Autodesk Inventor part; units mm, degrees
(part 3 of 4)
  line L545 (-44.5, 18.2583) -> (-43, 20.8564)
  line L546 (-59, 20.8564) -> (-60.5, 23.4545)
  line L547 (-60.5, 23.4545) -> (-63.5, 23.4545)
  line L548 (-63.5, 23.4545) -> (-65, 20.8564)
  line L549 (-65, 20.8564) -> (-63.5, 18.2583)
  line L550 (-63.5, 18.2583) -> (-60.5, 18.2583)
  line L551 (-60.5, 18.2583) -> (-59, 20.8564)
  line L552 (-75, 20.8564) -> (-76.5, 23.4545)
  line L553 (-76.5, 23.4545) -> (-79.5, 23.4545)
  line L554 (-79.5, 23.4545) -> (-81, 20.8564)
  line L555 (-81, 20.8564) -> (-79.5, 18.2583)
  line L556 (-79.5, 18.2583) -> (-76.5, 18.2583)
  line L557 (-76.5, 18.2583) -> (-75, 20.8564)
  line L558 (-80.5, 30.5263) -> (-83.5, 30.5263)
  line L559 (-83.5, 30.5263) -> (-85, 27.9282)
  line L560 (-85, 27.9282) -> (-83.5, 25.3301)
  line L561 (-83.5, 25.3301) -> (-80.5, 25.3301)
  line L562 (-80.5, 25.3301) -> (-79, 27.9282)
  line L563 (-79, 27.9282) -> (-80.5, 30.5263)
  line L564 (-47, 27.9282) -> (-48.5, 30.5263)
  line L565 (-48.5, 30.5263) -> (-51.5, 30.5263)
  line L566 (-51.5, 30.5263) -> (-53, 27.9282)
  line L567 (-53, 27.9282) -> (-51.5, 25.3301)
  line L568 (-51.5, 25.3301) -> (-48.5, 25.3301)
  line L569 (-48.5, 25.3301) -> (-47, 27.9282)
  line L570 (-67.5, 25.3301) -> (-64.5, 25.3301)
  line L571 (-64.5, 25.3301) -> (-63, 27.9282)
  line L572 (-63, 27.9282) -> (-64.5, 30.5263)
  line L573 (-64.5, 30.5263) -> (-67.5, 30.5263)
  line L574 (-67.5, 30.5263) -> (-69, 27.9282)
  line L575 (-69, 27.9282) -> (-67.5, 25.3301)
  line L576 (-39.5, 37.4545) -> (-41, 34.8564)
  line L577 (-41, 34.8564) -> (-39.5, 32.2583)
  line L578 (-39.5, 32.2583) -> (-36.5, 32.2583)
  line L579 (-36.5, 32.2583) -> (-35, 34.8564)
  line L580 (-35, 34.8564) -> (-36.5, 37.4545)
  line L581 (-36.5, 37.4545) -> (-39.5, 37.4545)
  line L582 (-55.5, 32.2583) -> (-52.5, 32.2583)
  line L583 (-52.5, 32.2583) -> (-51, 34.8564)
  line L584 (-51, 34.8564) -> (-52.5, 37.4545)
  line L585 (-52.5, 37.4545) -> (-55.5, 37.4545)
  line L586 (-55.5, 37.4545) -> (-57, 34.8564)
  line L587 (-57, 34.8564) -> (-55.5, 32.2583)
  line L588 (-71.5, 32.2583) -> (-68.5, 32.2583)
  line L589 (-68.5, 32.2583) -> (-67, 34.8564)
  line L590 (-67, 34.8564) -> (-68.5, 37.4545)
  line L591 (-68.5, 37.4545) -> (-71.5, 37.4545)
  line L592 (-71.5, 37.4545) -> (-73, 34.8564)
  line L593 (-73, 34.8564) -> (-71.5, 32.2583)
  line L594 (-15.5, 32.2583) -> (-12.5, 32.2583)
  line L595 (-12.5, 32.2583) -> (-11, 34.8564)
  line L596 (-11, 34.8564) -> (-12.5, 37.4545)
  line L597 (-12.5, 37.4545) -> (-15.5, 37.4545)
  line L598 (-15.5, 37.4545) -> (-17, 34.8564)
  line L599 (-17, 34.8564) -> (-15.5, 32.2583)
  line L600 (-35.5, 25.3301) -> (-32.5, 25.3301)
  line L601 (-32.5, 25.3301) -> (-31, 27.9282)
  line L602 (-31, 27.9282) -> (-32.5, 30.5263)
  line L603 (-32.5, 30.5263) -> (-35.5, 30.5263)
  line L604 (-35.5, 30.5263) -> (-37, 27.9282)
  line L605 (-37, 27.9282) -> (-35.5, 25.3301)
  line L606 (-25, 34.8564) -> (-23.5, 32.2583)
  line L607 (-23.5, 32.2583) -> (-20.5, 32.2583)
  line L608 (-20.5, 32.2583) -> (-19, 34.8564)
  line L609 (-19, 34.8564) -> (-20.5, 37.4545)
  line L610 (-20.5, 37.4545) -> (-23.5, 37.4545)
  line L611 (-23.5, 37.4545) -> (-25, 34.8564)
  line L612 (-7, 27.9282) -> (-8.5, 30.5263)
  line L613 (-8.5, 30.5263) -> (-11.5, 30.5263)
  line L614 (-11.5, 30.5263) -> (-13, 27.9282)
  line L615 (-13, 27.9282) -> (-11.5, 25.3301)
  line L616 (-11.5, 25.3301) -> (-8.5, 25.3301)
  line L617 (-8.5, 25.3301) -> (-7, 27.9282)
  line L618 (-80.5, 44.5263) -> (-83.5, 44.5263)
  line L619 (-83.5, 44.5263) -> (-85, 41.9282)
  line L620 (-85, 41.9282) -> (-83.5, 39.3301)
  line L621 (-83.5, 39.3301) -> (-80.5, 39.3301)
  line L622 (-80.5, 39.3301) -> (-79, 41.9282)
  line L623 (-79, 41.9282) -> (-80.5, 44.5263)
  line L624 (-47, 41.9282) -> (-48.5, 44.5263)
  line L625 (-48.5, 44.5263) -> (-51.5, 44.5263)
  line L626 (-51.5, 44.5263) -> (-53, 41.9282)
  line L627 (-53, 41.9282) -> (-51.5, 39.3301)
  line L628 (-51.5, 39.3301) -> (-48.5, 39.3301)
  line L629 (-48.5, 39.3301) -> (-47, 41.9282)
  line L630 (-67.5, 39.3301) -> (-64.5, 39.3301)
  line L631 (-64.5, 39.3301) -> (-63, 41.9282)
  line L632 (-63, 41.9282) -> (-64.5, 44.5263)
  line L633 (-64.5, 44.5263) -> (-67.5, 44.5263)
  line L634 (-67.5, 44.5263) -> (-69, 41.9282)
  line L635 (-69, 41.9282) -> (-67.5, 39.3301)
  line L636 (-39.5, 51.4545) -> (-41, 48.8564)
  line L637 (-41, 48.8564) -> (-39.5, 46.2583)
  line L638 (-39.5, 46.2583) -> (-36.5, 46.2583)
  line L639 (-36.5, 46.2583) -> (-35, 48.8564)
  line L640 (-35, 48.8564) -> (-36.5, 51.4545)
  line L641 (-36.5, 51.4545) -> (-39.5, 51.4545)
  line L642 (-55.5, 46.2583) -> (-52.5, 46.2583)
  line L643 (-52.5, 46.2583) -> (-51, 48.8564)
  line L644 (-51, 48.8564) -> (-52.5, 51.4545)
  line L645 (-52.5, 51.4545) -> (-55.5, 51.4545)
  line L646 (-55.5, 51.4545) -> (-57, 48.8564)
  line L647 (-57, 48.8564) -> (-55.5, 46.2583)
  line L648 (-71.5, 46.2583) -> (-68.5, 46.2583)
  line L649 (-68.5, 46.2583) -> (-67, 48.8564)
  line L650 (-67, 48.8564) -> (-68.5, 51.4545)
  line L651 (-68.5, 51.4545) -> (-71.5, 51.4545)
  line L652 (-71.5, 51.4545) -> (-73, 48.8564)
  line L653 (-73, 48.8564) -> (-71.5, 46.2583)
  line L654 (-15.5, 46.2583) -> (-12.5, 46.2583)
  line L655 (-12.5, 46.2583) -> (-11, 48.8564)
  line L656 (-11, 48.8564) -> (-12.5, 51.4545)
  line L657 (-12.5, 51.4545) -> (-15.5, 51.4545)
  line L658 (-15.5, 51.4545) -> (-17, 48.8564)
  line L659 (-17, 48.8564) -> (-15.5, 46.2583)
  line L660 (-35.5, 39.3301) -> (-32.5, 39.3301)
  line L661 (-32.5, 39.3301) -> (-31, 41.9282)
  line L662 (-31, 41.9282) -> (-32.5, 44.5263)
  line L663 (-32.5, 44.5263) -> (-35.5, 44.5263)
  line L664 (-35.5, 44.5263) -> (-37, 41.9282)
  line L665 (-37, 41.9282) -> (-35.5, 39.3301)
  line L666 (-25, 48.8564) -> (-23.5, 46.2583)
  line L667 (-23.5, 46.2583) -> (-20.5, 46.2583)
  line L668 (-20.5, 46.2583) -> (-19, 48.8564)
  line L669 (-19, 48.8564) -> (-20.5, 51.4545)
  line L670 (-20.5, 51.4545) -> (-23.5, 51.4545)
  line L671 (-23.5, 51.4545) -> (-25, 48.8564)
  line L672 (-7, 41.9282) -> (-8.5, 44.5263)
  line L673 (-8.5, 44.5263) -> (-11.5, 44.5263)
  line L674 (-11.5, 44.5263) -> (-13, 41.9282)
  line L675 (-13, 41.9282) -> (-11.5, 39.3301)
  line L676 (-11.5, 39.3301) -> (-8.5, 39.3301)
  line L677 (-8.5, 39.3301) -> (-7, 41.9282)
  line L678 (-80.5, 58.5263) -> (-83.5, 58.5263)
  line L679 (-83.5, 58.5263) -> (-85, 55.9282)
  line L680 (-85, 55.9282) -> (-83.5, 53.3301)
  line L681 (-83.5, 53.3301) -> (-80.5, 53.3301)
  line L682 (-80.5, 53.3301) -> (-79, 55.9282)
  line L683 (-79, 55.9282) -> (-80.5, 58.5263)
  line L684 (-47, 55.9282) -> (-48.5, 58.5263)
  line L685 (-48.5, 58.5263) -> (-51.5, 58.5263)
  line L686 (-51.5, 58.5263) -> (-53, 55.9282)
  line L687 (-53, 55.9282) -> (-51.5, 53.3301)
  line L688 (-51.5, 53.3301) -> (-48.5, 53.3301)
  line L689 (-48.5, 53.3301) -> (-47, 55.9282)
  line L690 (-67.5, 53.3301) -> (-64.5, 53.3301)
  line L691 (-64.5, 53.3301) -> (-63, 55.9282)
  line L692 (-63, 55.9282) -> (-64.5, 58.5263)
  line L693 (-64.5, 58.5263) -> (-67.5, 58.5263)
  line L694 (-67.5, 58.5263) -> (-69, 55.9282)
  line L695 (-69, 55.9282) -> (-67.5, 53.3301)
  line L696 (-39.5, 65.4545) -> (-41, 62.8564)
  line L697 (-41, 62.8564) -> (-39.5, 60.2583)
  line L698 (-39.5, 60.2583) -> (-36.5, 60.2583)
  line L699 (-36.5, 60.2583) -> (-35, 62.8564)
  line L700 (-35, 62.8564) -> (-36.5, 65.4545)
  line L701 (-36.5, 65.4545) -> (-39.5, 65.4545)
  line L702 (-55.5, 60.2583) -> (-52.5, 60.2583)
  line L703 (-52.5, 60.2583) -> (-51, 62.8564)
  line L704 (-51, 62.8564) -> (-52.5, 65.4545)
  line L705 (-52.5, 65.4545) -> (-55.5, 65.4545)
  line L706 (-55.5, 65.4545) -> (-57, 62.8564)
  line L707 (-57, 62.8564) -> (-55.5, 60.2583)
  line L708 (-71.5, 60.2583) -> (-68.5, 60.2583)
  line L709 (-68.5, 60.2583) -> (-67, 62.8564)
  line L710 (-67, 62.8564) -> (-68.5, 65.4545)
  line L711 (-68.5, 65.4545) -> (-71.5, 65.4545)
  line L712 (-71.5, 65.4545) -> (-73, 62.8564)
  line L713 (-73, 62.8564) -> (-71.5, 60.2583)
  line L714 (-15.5, 60.2583) -> (-12.5, 60.2583)
  line L715 (-12.5, 60.2583) -> (-11, 62.8564)
  line L716 (-11, 62.8564) -> (-12.5, 65.4545)
  line L717 (-12.5, 65.4545) -> (-15.5, 65.4545)
  line L718 (-15.5, 65.4545) -> (-17, 62.8564)
  line L719 (-17, 62.8564) -> (-15.5, 60.2583)
  line L720 (-35.5, 53.3301) -> (-32.5, 53.3301)
  line L721 (-32.5, 53.3301) -> (-31, 55.9282)
  line L722 (-31, 55.9282) -> (-32.5, 58.5263)
  line L723 (-32.5, 58.5263) -> (-35.5, 58.5263)
  line L724 (-35.5, 58.5263) -> (-37, 55.9282)
  line L725 (-37, 55.9282) -> (-35.5, 53.3301)
  line L726 (-25, 62.8564) -> (-23.5, 60.2583)
  line L727 (-23.5, 60.2583) -> (-20.5, 60.2583)
  line L728 (-20.5, 60.2583) -> (-19, 62.8564)
  line L729 (-19, 62.8564) -> (-20.5, 65.4545)
  line L730 (-20.5, 65.4545) -> (-23.5, 65.4545)
  line L731 (-23.5, 65.4545) -> (-25, 62.8564)
  line L732 (-7, 55.9282) -> (-8.5, 58.5263)
  line L733 (-8.5, 58.5263) -> (-11.5, 58.5263)
  line L734 (-11.5, 58.5263) -> (-13, 55.9282)
  line L735 (-13, 55.9282) -> (-11.5, 53.3301)
  line L736 (-11.5, 53.3301) -> (-8.5, 53.3301)
  line L737 (-8.5, 53.3301) -> (-7, 55.9282)
  line L738 (-80.5, 72.5263) -> (-83.5, 72.5263)
  line L739 (-83.5, 72.5263) -> (-85, 69.9282)
  line L740 (-85, 69.9282) -> (-83.5, 67.3301)
  line L741 (-83.5, 67.3301) -> (-80.5, 67.3301)
  line L742 (-80.5, 67.3301) -> (-79, 69.9282)
  line L743 (-79, 69.9282) -> (-80.5, 72.5263)
  line L744 (-47, 69.9282) -> (-48.5, 72.5263)
  line L745 (-48.5, 72.5263) -> (-51.5, 72.5263)
  line L746 (-51.5, 72.5263) -> (-53, 69.9282)
  line L747 (-53, 69.9282) -> (-51.5, 67.3301)
  line L748 (-51.5, 67.3301) -> (-48.5, 67.3301)
  line L749 (-48.5, 67.3301) -> (-47, 69.9282)
  line L750 (-67.5, 67.3301) -> (-64.5, 67.3301)
  line L751 (-64.5, 67.3301) -> (-63, 69.9282)
  line L752 (-63, 69.9282) -> (-64.5, 72.5263)
  line L753 (-64.5, 72.5263) -> (-67.5, 72.5263)
  line L754 (-67.5, 72.5263) -> (-69, 69.9282)
  line L755 (-69, 69.9282) -> (-67.5, 67.3301)
  line L756 (-39.5, 79.4545) -> (-41, 76.8564)
  line L757 (-41, 76.8564) -> (-39.5, 74.2583)
  line L758 (-39.5, 74.2583) -> (-36.5, 74.2583)
  line L759 (-36.5, 74.2583) -> (-35, 76.8564)
  line L760 (-35, 76.8564) -> (-36.5, 79.4545)
  line L761 (-36.5, 79.4545) -> (-39.5, 79.4545)
  line L762 (-55.5, 74.2583) -> (-52.5, 74.2583)
  line L763 (-52.5, 74.2583) -> (-51, 76.8564)
  line L764 (-51, 76.8564) -> (-52.5, 79.4545)
  line L765 (-52.5, 79.4545) -> (-55.5, 79.4545)
  line L766 (-55.5, 79.4545) -> (-57, 76.8564)
  line L767 (-57, 76.8564) -> (-55.5, 74.2583)
  line L768 (-71.5, 74.2583) -> (-68.5, 74.2583)
  line L769 (-68.5, 74.2583) -> (-67, 76.8564)
  line L770 (-67, 76.8564) -> (-68.5, 79.4545)
  line L771 (-68.5, 79.4545) -> (-71.5, 79.4545)
  line L772 (-71.5, 79.4545) -> (-73, 76.8564)
  line L773 (-73, 76.8564) -> (-71.5, 74.2583)
  line L774 (-15.5, 74.2583) -> (-12.5, 74.2583)
  line L775 (-12.5, 74.2583) -> (-11, 76.8564)
  line L776 (-11, 76.8564) -> (-12.5, 79.4545)
  line L777 (-12.5, 79.4545) -> (-15.5, 79.4545)
  line L778 (-15.5, 79.4545) -> (-17, 76.8564)
  line L779 (-17, 76.8564) -> (-15.5, 74.2583)
  line L780 (-35.5, 67.3301) -> (-32.5, 67.3301)
  line L781 (-32.5, 67.3301) -> (-31, 69.9282)
  line L782 (-31, 69.9282) -> (-32.5, 72.5263)
  line L783 (-32.5, 72.5263) -> (-35.5, 72.5263)
  line L784 (-35.5, 72.5263) -> (-37, 69.9282)
  line L785 (-37, 69.9282) -> (-35.5, 67.3301)
  line L786 (-25, 76.8564) -> (-23.5, 74.2583)
  line L787 (-23.5, 74.2583) -> (-20.5, 74.2583)
  line L788 (-20.5, 74.2583) -> (-19, 76.8564)
  line L789 (-19, 76.8564) -> (-20.5, 79.4545)
  line L790 (-20.5, 79.4545) -> (-23.5, 79.4545)
  line L791 (-23.5, 79.4545) -> (-25, 76.8564)
  line L792 (-7, 69.9282) -> (-8.5, 72.5263)
  line L793 (-8.5, 72.5263) -> (-11.5, 72.5263)
  line L794 (-11.5, 72.5263) -> (-13, 69.9282)
  line L795 (-13, 69.9282) -> (-11.5, 67.3301)
  line L796 (-11.5, 67.3301) -> (-8.5, 67.3301)
  line L797 (-8.5, 67.3301) -> (-7, 69.9282)
  line L798 (-80.5, 86.5263) -> (-83.5, 86.5263)
  line L799 (-83.5, 86.5263) -> (-85, 83.9282)
  line L800 (-85, 83.9282) -> (-83.5, 81.3301)
  line L801 (-83.5, 81.3301) -> (-80.5, 81.3301)
  line L802 (-80.5, 81.3301) -> (-79, 83.9282)
  line L803 (-79, 83.9282) -> (-80.5, 86.5263)
  line L804 (-47, 83.9282) -> (-48.5, 86.5263)
  line L805 (-48.5, 86.5263) -> (-51.5, 86.5263)
  line L806 (-51.5, 86.5263) -> (-53, 83.9282)
  line L807 (-53, 83.9282) -> (-51.5, 81.3301)
  line L808 (-51.5, 81.3301) -> (-48.5, 81.3301)
  line L809 (-48.5, 81.3301) -> (-47, 83.9282)
  line L810 (-67.5, 81.3301) -> (-64.5, 81.3301)
  line L811 (-64.5, 81.3301) -> (-63, 83.9282)
  line L812 (-63, 83.9282) -> (-64.5, 86.5263)
  line L813 (-64.5, 86.5263) -> (-67.5, 86.5263)
  line L814 (-67.5, 86.5263) -> (-69, 83.9282)
  line L815 (-69, 83.9282) -> (-67.5, 81.3301)
  line L816 (-39.5, 93.4545) -> (-41, 90.8564)
  line L817 (-41, 90.8564) -> (-39.5, 88.2583)
  line L818 (-39.5, 88.2583) -> (-36.5, 88.2583)
  line L819 (-36.5, 88.2583) -> (-35, 90.8564)
  line L820 (-35, 90.8564) -> (-36.5, 93.4545)
  line L821 (-36.5, 93.4545) -> (-39.5, 93.4545)
  line L822 (-55.5, 88.2583) -> (-52.5, 88.2583)
  line L823 (-52.5, 88.2583) -> (-51, 90.8564)
  line L824 (-51, 90.8564) -> (-52.5, 93.4545)
  line L825 (-52.5, 93.4545) -> (-55.5, 93.4545)
  line L826 (-55.5, 93.4545) -> (-57, 90.8564)
  line L827 (-57, 90.8564) -> (-55.5, 88.2583)
  line L828 (-71.5, 88.2583) -> (-68.5, 88.2583)
  line L829 (-68.5, 88.2583) -> (-67, 90.8564)
  line L830 (-67, 90.8564) -> (-68.5, 93.4545)
  line L831 (-68.5, 93.4545) -> (-71.5, 93.4545)
  line L832 (-71.5, 93.4545) -> (-73, 90.8564)
  line L833 (-73, 90.8564) -> (-71.5, 88.2583)
  line L834 (-27.5, 81.3301) -> (-24.5, 81.3301)
  line L835 (-24.5, 81.3301) -> (-23, 83.9282)
  line L836 (-23, 83.9282) -> (-24.5, 86.5263)
  line L837 (-24.5, 86.5263) -> (-27.5, 86.5263)
  line L838 (-27.5, 86.5263) -> (-29, 83.9282)
  line L839 (-29, 83.9282) -> (-27.5, 81.3301)
  line L840 (-19.5, 86.5263) -> (-21, 83.9282)
  line L841 (-21, 83.9282) -> (-19.5, 81.3301)
  line L842 (-19.5, 81.3301) -> (-16.5, 81.3301)
  line L843 (-16.5, 81.3301) -> (-15, 83.9282)
  line L844 (-15, 83.9282) -> (-16.5, 86.5263)
  line L845 (-16.5, 86.5263) -> (-19.5, 86.5263)
  line L846 (-80.5, 100.5263) -> (-83.5, 100.5263)
  line L847 (-83.5, 100.5263) -> (-85, 97.9282)
  line L848 (-85, 97.9282) -> (-83.5, 95.3301)
  line L849 (-83.5, 95.3301) -> (-80.5, 95.3301)
  line L850 (-80.5, 95.3301) -> (-79, 97.9282)
  line L851 (-79, 97.9282) -> (-80.5, 100.5263)
  line L852 (-47, 97.9282) -> (-48.5, 100.5263)
  line L853 (-48.5, 100.5263) -> (-51.5, 100.5263)
  line L854 (-51.5, 100.5263) -> (-53, 97.9282)
  line L855 (-53, 97.9282) -> (-51.5, 95.3301)
  line L856 (-51.5, 95.3301) -> (-48.5, 95.3301)
  line L857 (-48.5, 95.3301) -> (-47, 97.9282)
  line L858 (-67.5, 95.3301) -> (-64.5, 95.3301)
  line L859 (-64.5, 95.3301) -> (-63, 97.9282)
  line L860 (-63, 97.9282) -> (-64.5, 100.5263)
  line L861 (-64.5, 100.5263) -> (-67.5, 100.5263)
  line L862 (-67.5, 100.5263) -> (-69, 97.9282)
  line L863 (-69, 97.9282) -> (-67.5, 95.3301)
  line L864 (-39.5, 107.4545) -> (-41, 104.8564)
  line L865 (-41, 104.8564) -> (-39.5, 102.2583)
  line L866 (-39.5, 102.2583) -> (-36.5, 102.2583)
  line L867 (-36.5, 102.2583) -> (-35, 104.8564)
  line L868 (-35, 104.8564) -> (-36.5, 107.4545)
  line L869 (-36.5, 107.4545) -> (-39.5, 107.4545)
  line L870 (-55.5, 102.2583) -> (-52.5, 102.2583)
  line L871 (-52.5, 102.2583) -> (-51, 104.8564)
  line L872 (-51, 104.8564) -> (-52.5, 107.4545)
  line L873 (-52.5, 107.4545) -> (-55.5, 107.4545)
  line L874 (-55.5, 107.4545) -> (-57, 104.8564)
  line L875 (-57, 104.8564) -> (-55.5, 102.2583)
  line L876 (-71.5, 102.2583) -> (-68.5, 102.2583)
  line L877 (-68.5, 102.2583) -> (-67, 104.8564)
  line L878 (-67, 104.8564) -> (-68.5, 107.4545)
  line L879 (-68.5, 107.4545) -> (-71.5, 107.4545)
  line L880 (-71.5, 107.4545) -> (-73, 104.8564)
  line L881 (-73, 104.8564) -> (-71.5, 102.2583)
  line L882 (-35.5, 95.3301) -> (-32.5, 95.3301)
  line L883 (-32.5, 95.3301) -> (-31, 97.9282)
  line L884 (-31, 97.9282) -> (-32.5, 100.5263)
  line L885 (-32.5, 100.5263) -> (-35.5, 100.5263)
  line L886 (-35.5, 100.5263) -> (-37, 97.9282)
  line L887 (-37, 97.9282) -> (-35.5, 95.3301)
  line L888 (-71, 111.9282) -> (-72.5, 114.5263)
  line L889 (-72.5, 114.5263) -> (-75.5, 114.5263)
  line L890 (-75.5, 114.5263) -> (-77, 111.9282)
  line L891 (-77, 111.9282) -> (-75.5, 109.3301)
  line L892 (-75.5, 109.3301) -> (-72.5, 109.3301)
  line L893 (-72.5, 109.3301) -> (-71, 111.9282)
  line L894 (-59.5, 109.3301) -> (-56.5, 109.3301)
  line L895 (-56.5, 109.3301) -> (-55, 111.9282)
  line L896 (-55, 111.9282) -> (-56.5, 114.5263)
  line L897 (-56.5, 114.5263) -> (-59.5, 114.5263)
  line L898 (-59.5, 114.5263) -> (-61, 111.9282)
  line L899 (-61, 111.9282) -> (-59.5, 109.3301)
  line L900 (-79.5, 121.4545) -> (-81, 118.8564)
  line L901 (-81, 118.8564) -> (-79.5, 116.2583)
  line L902 (-79.5, 116.2583) -> (-76.5, 116.2583)
  line L903 (-76.5, 116.2583) -> (-75, 118.8564)
  line L904 (-75, 118.8564) -> (-76.5, 121.4545)
  line L905 (-76.5, 121.4545) -> (-79.5, 121.4545)
  line L906 (-47.5, 116.2583) -> (-44.5, 116.2583)
  line L907 (-44.5, 116.2583) -> (-43, 118.8564)
  line L908 (-43, 118.8564) -> (-44.5, 121.4545)
  line L909 (-44.5, 121.4545) -> (-47.5, 121.4545)
  line L910 (-47.5, 121.4545) -> (-49, 118.8564)
  line L911 (-49, 118.8564) -> (-47.5, 116.2583)
  line L912 (-63.5, 116.2583) -> (-60.5, 116.2583)
  line L913 (-60.5, 116.2583) -> (-59, 118.8564)
  line L914 (-59, 118.8564) -> (-60.5, 121.4545)
  line L915 (-60.5, 121.4545) -> (-63.5, 121.4545)
  line L916 (-63.5, 121.4545) -> (-65, 118.8564)
  line L917 (-65, 118.8564) -> (-63.5, 116.2583)
  line L918 (-39, 111.9282) -> (-40.5, 114.5263)
  line L919 (-40.5, 114.5263) -> (-43.5, 114.5263)
  line L920 (-43.5, 114.5263) -> (-45, 111.9282)
  line L921 (-45, 111.9282) -> (-43.5, 109.3301)
  line L922 (-43.5, 109.3301) -> (-40.5, 109.3301)
  line L923 (-40.5, 109.3301) -> (-39, 111.9282)
  line L924 (-80.5, 128.5263) -> (-83.5, 128.5263)
  line L925 (-83.5, 128.5263) -> (-85, 125.9282)
  line L926 (-85, 125.9282) -> (-83.5, 123.3301)
  line L927 (-83.5, 123.3301) -> (-80.5, 123.3301)
  line L928 (-80.5, 123.3301) -> (-79, 125.9282)
  line L929 (-79, 125.9282) -> (-80.5, 128.5263)
  line L930 (-47, 125.9282) -> (-48.5, 128.5263)
  line L931 (-48.5, 128.5263) -> (-51.5, 128.5263)
  line L932 (-51.5, 128.5263) -> (-53, 125.9282)
  line L933 (-53, 125.9282) -> (-51.5, 123.3301)
  line L934 (-51.5, 123.3301) -> (-48.5, 123.3301)
  line L935 (-48.5, 123.3301) -> (-47, 125.9282)
  line L936 (-67.5, 123.3301) -> (-64.5, 123.3301)
  line L937 (-64.5, 123.3301) -> (-63, 125.9282)
  line L938 (-63, 125.9282) -> (-64.5, 128.5263)
  line L939 (-64.5, 128.5263) -> (-67.5, 128.5263)
  line L940 (-67.5, 128.5263) -> (-69, 125.9282)
  line L941 (-69, 125.9282) -> (-67.5, 123.3301)
  line L942 (-39.5, 135.4545) -> (-41, 132.8564)
  line L943 (-41, 132.8564) -> (-39.5, 130.2583)
  line L944 (-39.5, 130.2583) -> (-36.5, 130.2583)
  line L945 (-36.5, 130.2583) -> (-35, 132.8564)
  line L946 (-35, 132.8564) -> (-36.5, 135.4545)
  line L947 (-36.5, 135.4545) -> (-39.5, 135.4545)
  line L948 (-55.5, 130.2583) -> (-52.5, 130.2583)
  line L949 (-52.5, 130.2583) -> (-51, 132.8564)
  line L950 (-51, 132.8564) -> (-52.5, 135.4545)
  line L951 (-52.5, 135.4545) -> (-55.5, 135.4545)
  line L952 (-55.5, 135.4545) -> (-57, 132.8564)
  line L953 (-57, 132.8564) -> (-55.5, 130.2583)
  line L954 (-71.5, 130.2583) -> (-68.5, 130.2583)
  line L955 (-68.5, 130.2583) -> (-67, 132.8564)
  line L956 (-67, 132.8564) -> (-68.5, 135.4545)
  line L957 (-68.5, 135.4545) -> (-71.5, 135.4545)
  line L958 (-71.5, 135.4545) -> (-73, 132.8564)
  line L959 (-73, 132.8564) -> (-71.5, 130.2583)
  line L960 (-35.5, 123.3301) -> (-32.5, 123.3301)
  line L961 (-32.5, 123.3301) -> (-31, 125.9282)
  line L962 (-31, 125.9282) -> (-32.5, 128.5263)
  line L963 (-32.5, 128.5263) -> (-35.5, 128.5263)
  line L964 (-35.5, 128.5263) -> (-37, 125.9282)
  line L965 (-37, 125.9282) -> (-35.5, 123.3301)
  line L966 (-86, 150) -> (0, 150)
  line L967 (0, 150) -> (0, 0)
  line L968 (0, 0) -> (-86, 0)
  line L969 (-86, 0) -> (-86, 150)
  line L970 (-24.5, 100.7272) -> (-11.5, 100.7272) construction
  line L971 (-11.5, 100.7272) -> (-11.5, 125.7272)
  line L972 (-11.5, 125.7272) -> (-24.5, 125.7272) construction
  line L973 (-24.5, 125.7272) -> (-24.5, 100.7272)
  line L974 (-24.5, 100.7272) -> (-11.5, 125.7272) construction
  line L975 (-11.5, 100.7272) -> (-24.5, 125.7272) construction
  line L976 (-18, 100.7272) -> (-18, 90.7272) construction
  line L977 (-18, 90.7272) -> (-24.5, 100.7272)
  line L978 (-18, 90.7272) -> (-11.5, 100.7272)
  line L979 (-24.5, 113.2272) -> (-11.5, 113.2272) construction
  line L980 (-18, 125.7272) -> (-18, 135.7272) construction
  line L981 (-18, 135.7272) -> (-24.5, 125.7272)
  line L982 (-18, 135.7272) -> (-11.5, 125.7272)
  line L983 (-14.75, 112.2272) -> (-21.25, 112.2272)
  line L984 (-21.25, 112.2272) -> (-21.25, 114.2272)
  line L985 (-21.25, 114.2272) -> (-14.75, 114.2272)
  line L986 (-14.75, 114.2272) -> (-14.75, 112.2272)
  line L987 (-14.75, 112.2272) -> (-21.25, 114.2272) construction
  line L988 (-21.25, 112.2272) -> (-14.75, 114.2272) construction
  line L989 (-21.25, 119.2272) -> (-14.75, 119.2272)
  line L990 (-21.25, 117.2272) -> (-21.25, 119.2272)
  line L991 (-14.75, 119.2272) -> (-14.75, 117.2272)
  line L992 (-14.75, 117.2272) -> (-21.25, 119.2272) construction
  line L993 (-21.25, 117.2272) -> (-14.75, 119.2272) construction
  line L994 (-14.75, 117.2272) -> (-21.25, 117.2272)
  line L995 (-21.25, 109.2272) -> (-14.75, 109.2272)
  line L996 (-14.75, 109.2272) -> (-14.75, 107.2272)
  line L997 (-14.75, 107.2272) -> (-21.25, 107.2272)
  line L998 (-14.75, 107.2272) -> (-21.25, 109.2272) construction
  line L999 (-21.25, 107.2272) -> (-14.75, 109.2272) construction
  line L1000 (-21.25, 107.2272) -> (-21.25, 109.2272)
  line L1001 (-23, 101.1719) -> (-23, 125.2826)
  line L1002 (-23, 125.2826) -> (-18, 132.9749)
  line L1003 (-18, 132.9749) -> (-13, 125.2826)
  line L1004 (-13, 125.2826) -> (-13, 101.1719)
  line L1005 (-13, 101.1719) -> (-18, 93.4796)
  line L1006 (-18, 93.4796) -> (-23, 101.1719)
  line L1007 (-22, 109.9772) -> (-22, 106.4772)
  line L1008 (-22, 106.4772) -> (-14, 106.4772)
  line L1009 (-14, 106.4772) -> (-14, 109.9772)
  line L1010 (-14, 109.9772) -> (-22, 109.9772)
  line L1011 (-22, 114.9772) -> (-22, 111.4772)
  line L1012 (-22, 111.4772) -> (-14, 111.4772)
  line L1013 (-14, 111.4772) -> (-14, 114.9772)
  line L1014 (-14, 114.9772) -> (-22, 114.9772)
  line L1015 (-22, 119.9772) -> (-22, 116.4772)
  line L1016 (-22, 116.4772) -> (-14, 116.4772)
  line L1017 (-14, 116.4772) -> (-14, 119.9772)
  line L1018 (-14, 119.9772) -> (-22, 119.9772)
  line L1019 (-25.3156, 100.4855) -> (-25.3156, 125.969)
  line L1020 (-25.3156, 125.969) -> (-18, 137.2237)
  line L1021 (-18, 137.2237) -> (-10.6844, 125.969)
  line L1022 (-10.6844, 125.969) -> (-10.6844, 100.4855)
  line L1023 (-10.6844, 100.4855) -> (-18, 89.2308)
  line L1024 (-18, 89.2308) -> (-25.3156, 100.4855)
  point P0 (0, 75)
  point P1 (-18, 113.2272)
  point P2 (-18, 118.2272)
  point P3 (-18, 108.2272)
  dimension "d49" = 13
  dimension "d50" = 25
  dimension "d51" = 10
  dimension "d52" = 2
  dimension "d55" = 5
  dimension "d62" = 5
  dimension "d67" = 0.8156
  constraints: 110 end point, 11 midpoint, 8 parallel, 3 perpendicular, 3 vertical, 2 collinear, 2 symmetric about line, 1 horizontal, 39 other
  measures "d49" distance of L972.end L971.end
  measures "d50" distance of L971.end L970.end
  measures "d51" distance of L976.start L976.end
  measures "d52" distance of L983.end L984.end
  measures "d55" distance of L984.end L989.start
  measures "d62" distance of L984.end L995.start
  measures "d67" distance between parallel lines of L977 L1024
extrude "Estrusione5" cut sketch "Schizzo6" against normal blind 1 contours L1001 L1002 L1003 L1004 L1005 L1006 | L1019 L1020 L1021 L1022 L1023 L1024
sketch "Schizzo7" plane through (70, 25.7272, 11.5) normal (1, 0, 0) x (0, 0, -1)
  line L0 (-13, 0) -> (-6.5, -10)
  line L1 (-6.5, -10) -> (0, 0)
  line L2 (0, 0) -> (0, 25)
  line L3 (0, 25) -> (-6.5, 35)
  line L4 (-6.5, 35) -> (-13, 25)
  line L5 (-13, 25) -> (-13, 0)
  line L6 (-6.5, -7.2476) -> (-11.5, 0.4447)
  line L7 (-11.5, 0.4447) -> (-11.5, 24.5553)
  line L8 (-11.5, 24.5553) -> (-6.5, 32.2476)
  line L9 (-6.5, 32.2476) -> (-1.5, 24.5553)
  line L10 (-1.5, 24.5553) -> (-1.5, 0.4447)
  line L11 (-1.5, 0.4447) -> (-6.5, -7.2476)
  line L12 (-10.5, 5.75) -> (-2.5, 5.75)
  line L13 (-2.5, 5.75) -> (-2.5, 9.25)
  line L14 (-2.5, 9.25) -> (-10.5, 9.25)
  line L15 (-10.5, 9.25) -> (-10.5, 5.75)
  line L16 (-10.5, 10.75) -> (-2.5, 10.75)
  line L17 (-2.5, 10.75) -> (-2.5, 14.25)
  line L18 (-2.5, 14.25) -> (-10.5, 14.25)
  line L19 (-10.5, 14.25) -> (-10.5, 10.75)
  line L20 (-10.5, 15.75) -> (-2.5, 15.75)
  line L21 (-2.5, 15.75) -> (-2.5, 19.25)
  line L22 (-2.5, 19.25) -> (-10.5, 19.25)
  line L23 (-10.5, 19.25) -> (-10.5, 15.75)
  line L24 (-10, 6.25) -> (-3, 6.25)
  line L25 (-3, 6.25) -> (-3, 8.75)
  line L26 (-3, 8.75) -> (-10, 8.75)
  line L27 (-10, 8.75) -> (-10, 6.25)
  line L28 (-10, 11.25) -> (-3, 11.25)
  line L29 (-3, 11.25) -> (-3, 13.75)
  line L30 (-3, 13.75) -> (-10, 13.75)
  line L31 (-10, 13.75) -> (-10, 11.25)
  line L32 (-10, 16.25) -> (-3, 16.25)
  line L33 (-3, 16.25) -> (-3, 18.75)
  line L34 (-3, 18.75) -> (-10, 18.75)
  line L35 (-10, 18.75) -> (-10, 16.25)
  point P0 (11.5, -25.7272)
  constraints: 24 end point, 9 other
extrude "Estrusione6" add sketch "Schizzo7" along normal blind 4 contours L5 L4 L3 L2 L1 L0 | L27 L26 L25 L24 | L31 L30 L29 L28 | L35 L34 L33 L32
sketch "Schizzo8" plane through (-70, -75, 0) normal (-1, 0, 0) x (0, 0, 1)
  line L0 (0, 150) -> (86, 150)
  line L1 (86, 150) -> (86, 0)
  line L2 (86, 0) -> (0, 0)
  line L3 (0, 0) -> (0, 150)
  circle A0 centre (67.5127, 129.708) radius 15
  circle A1 centre (67.5127, 129.708) radius 13.3417
  point P0 (0, 75)
  dimension "d72" = 30
  dimension "d73" = 1.6583
  constraints: 2 centre point
  measures "d72" diameter of A0
  measures "d73" radial gap between concentric circles of A0 A1
extrude "Estrusione7" add sketch "Schizzo8" along normal blind 2 contours A0
sketch "Schizzo9" plane through (-70, 54.708, 67.5127) normal (-1, 0, 0) x (0, 0, 1)
  circle A0 centre (0, 0) radius 13.3417
  circle A1 centre (0, 0) radius 15
  line L0 (-67.5127, 20.292) -> (18.4873, 20.292)
  line L1 (18.4873, 20.292) -> (18.4873, -129.708)
  line L2 (18.4873, -129.708) -> (-67.5127, -129.708)
  line L3 (-67.5127, -129.708) -> (-67.5127, 20.292)
  point P0 (-67.5127, -54.708)
extrude "Estrusione8" cut sketch "Schizzo9" against normal blind 5 contours A0
sketch "Schizzo10" plane through (70, -75, 0) normal (1, 0, 0) x (0, 0, -1)
  line L0 (-18, 89.2308) -> (-25.3156, 100.4855)
  line L1 (-25.3156, 100.4855) -> (-25.3156, 125.969)
  line L2 (-25.3156, 125.969) -> (-18, 137.2237)
  line L3 (-18, 137.2237) -> (-10.6844, 125.969)
  line L4 (-10.6844, 125.969) -> (-10.6844, 100.4855)
  line L5 (-10.6844, 100.4855) -> (-18, 89.2308)
  line L6 (-43.5, 123.3301) -> (-45, 125.9282)
  line L7 (-45, 125.9282) -> (-43.5, 128.5263)
  line L8 (-43.5, 128.5263) -> (-40.5, 128.5263)
  line L9 (-40.5, 128.5263) -> (-39, 125.9282)
  line L10 (-39, 125.9282) -> (-40.5, 123.3301)
  line L11 (-40.5, 123.3301) -> (-43.5, 123.3301)
  line L12 (-63.5, 135.4545) -> (-60.5, 135.4545)
  line L13 (-60.5, 135.4545) -> (-59, 132.8564)
  line L14 (-59, 132.8564) -> (-60.5, 130.2583)
  line L15 (-60.5, 130.2583) -> (-63.5, 130.2583)
  line L16 (-63.5, 130.2583) -> (-65, 132.8564)
  line L17 (-65, 132.8564) -> (-63.5, 135.4545)
  line L18 (-47.5, 135.4545) -> (-44.5, 135.4545)
  line L19 (-44.5, 135.4545) -> (-43, 132.8564)
  line L20 (-43, 132.8564) -> (-44.5, 130.2583)
  line L21 (-44.5, 130.2583) -> (-47.5, 130.2583)
  line L22 (-47.5, 130.2583) -> (-49, 132.8564)
  line L23 (-49, 132.8564) -> (-47.5, 135.4545)
  line L24 (-59.5, 128.5263) -> (-56.5, 128.5263)
  line L25 (-56.5, 128.5263) -> (-55, 125.9282)
  line L26 (-55, 125.9282) -> (-56.5, 123.3301)
  line L27 (-56.5, 123.3301) -> (-59.5, 123.3301)
  line L28 (-59.5, 123.3301) -> (-61, 125.9282)
  line L29 (-61, 125.9282) -> (-59.5, 128.5263)
  line L30 (-75.5, 123.3301) -> (-77, 125.9282)
  line L31 (-77, 125.9282) -> (-75.5, 128.5263)
  line L32 (-75.5, 128.5263) -> (-72.5, 128.5263)
  line L33 (-72.5, 128.5263) -> (-71, 125.9282)
  line L34 (-71, 125.9282) -> (-72.5, 123.3301)
  line L35 (-72.5, 123.3301) -> (-75.5, 123.3301)
  line L36 (-35.5, 114.5263) -> (-32.5, 114.5263)
  line L37 (-32.5, 114.5263) -> (-31, 111.9282)
  line L38 (-31, 111.9282) -> (-32.5, 109.3301)
  line L39 (-32.5, 109.3301) -> (-35.5, 109.3301)
  line L40 (-35.5, 109.3301) -> (-37, 111.9282)
  line L41 (-37, 111.9282) -> (-35.5, 114.5263)
  line L42 (-71.5, 121.4545) -> (-68.5, 121.4545)
  line L43 (-68.5, 121.4545) -> (-67, 118.8564)
  line L44 (-67, 118.8564) -> (-68.5, 116.2583)
  line L45 (-68.5, 116.2583) -> (-71.5, 116.2583)
  line L46 (-71.5, 116.2583) -> (-73, 118.8564)
  line L47 (-73, 118.8564) -> (-71.5, 121.4545)
  line L48 (-55.5, 121.4545) -> (-52.5, 121.4545)
  line L49 (-52.5, 121.4545) -> (-51, 118.8564)
  line L50 (-51, 118.8564) -> (-52.5, 116.2583)
  line L51 (-52.5, 116.2583) -> (-55.5, 116.2583)
  line L52 (-55.5, 116.2583) -> (-57, 118.8564)
  line L53 (-57, 118.8564) -> (-55.5, 121.4545)
  line L54 (-35, 118.8564) -> (-36.5, 116.2583)
  line L55 (-36.5, 116.2583) -> (-39.5, 116.2583)
  line L56 (-39.5, 116.2583) -> (-41, 118.8564)
  line L57 (-41, 118.8564) -> (-39.5, 121.4545)
  line L58 (-39.5, 121.4545) -> (-36.5, 121.4545)
  line L59 (-36.5, 121.4545) -> (-35, 118.8564)
  line L60 (-67.5, 114.5263) -> (-64.5, 114.5263)
  line L61 (-64.5, 114.5263) -> (-63, 111.9282)
  line L62 (-63, 111.9282) -> (-64.5, 109.3301)
  line L63 (-64.5, 109.3301) -> (-67.5, 109.3301)
  line L64 (-67.5, 109.3301) -> (-69, 111.9282)
  line L65 (-69, 111.9282) -> (-67.5, 114.5263)
  line L66 (-51.5, 109.3301) -> (-53, 111.9282)
  line L67 (-53, 111.9282) -> (-51.5, 114.5263)
  line L68 (-51.5, 114.5263) -> (-48.5, 114.5263)
  line L69 (-48.5, 114.5263) -> (-47, 111.9282)
  line L70 (-47, 111.9282) -> (-48.5, 109.3301)
  line L71 (-48.5, 109.3301) -> (-51.5, 109.3301)
  line L72 (-80.5, 114.5263) -> (-79, 111.9282)
  line L73 (-79, 111.9282) -> (-80.5, 109.3301)
  line L74 (-80.5, 109.3301) -> (-83.5, 109.3301)
  line L75 (-83.5, 109.3301) -> (-85, 111.9282)
  line L76 (-85, 111.9282) -> (-83.5, 114.5263)
  line L77 (-83.5, 114.5263) -> (-80.5, 114.5263)
  line L78 (-43.5, 95.3301) -> (-45, 97.9282)
  line L79 (-45, 97.9282) -> (-43.5, 100.5263)
  line L80 (-43.5, 100.5263) -> (-40.5, 100.5263)
  line L81 (-40.5, 100.5263) -> (-39, 97.9282)
  line L82 (-39, 97.9282) -> (-40.5, 95.3301)
  line L83 (-40.5, 95.3301) -> (-43.5, 95.3301)
  line L84 (-63.5, 107.4545) -> (-60.5, 107.4545)
  line L85 (-60.5, 107.4545) -> (-59, 104.8564)
  line L86 (-59, 104.8564) -> (-60.5, 102.2583)
  line L87 (-60.5, 102.2583) -> (-63.5, 102.2583)
  line L88 (-63.5, 102.2583) -> (-65, 104.8564)
  line L89 (-65, 104.8564) -> (-63.5, 107.4545)
  line L90 (-47.5, 107.4545) -> (-44.5, 107.4545)
  line L91 (-44.5, 107.4545) -> (-43, 104.8564)
  line L92 (-43, 104.8564) -> (-44.5, 102.2583)
  line L93 (-44.5, 102.2583) -> (-47.5, 102.2583)
  line L94 (-47.5, 102.2583) -> (-49, 104.8564)
  line L95 (-49, 104.8564) -> (-47.5, 107.4545)
  line L96 (-75, 104.8564) -> (-76.5, 102.2583)
  line L97 (-76.5, 102.2583) -> (-79.5, 102.2583)
  line L98 (-79.5, 102.2583) -> (-81, 104.8564)
  line L99 (-81, 104.8564) -> (-79.5, 107.4545)
  line L100 (-79.5, 107.4545) -> (-76.5, 107.4545)
  line L101 (-76.5, 107.4545) -> (-75, 104.8564)
  line L102 (-59.5, 100.5263) -> (-56.5, 100.5263)
  line L103 (-56.5, 100.5263) -> (-55, 97.9282)
  line L104 (-55, 97.9282) -> (-56.5, 95.3301)
  line L105 (-56.5, 95.3301) -> (-59.5, 95.3301)
  line L106 (-59.5, 95.3301) -> (-61, 97.9282)
  line L107 (-61, 97.9282) -> (-59.5, 100.5263)
  line L108 (-75.5, 95.3301) -> (-77, 97.9282)
  line L109 (-77, 97.9282) -> (-75.5, 100.5263)
  line L110 (-75.5, 100.5263) -> (-72.5, 100.5263)
  line L111 (-72.5, 100.5263) -> (-71, 97.9282)
  line L112 (-71, 97.9282) -> (-72.5, 95.3301)
  line L113 (-72.5, 95.3301) -> (-75.5, 95.3301)
  line L114 (-11.5, 81.3301) -> (-13, 83.9282)
  line L115 (-13, 83.9282) -> (-11.5, 86.5263)
  line L116 (-11.5, 86.5263) -> (-8.5, 86.5263)
  line L117 (-8.5, 86.5263) -> (-7, 83.9282)
  line L118 (-7, 83.9282) -> (-8.5, 81.3301)
  line L119 (-8.5, 81.3301) -> (-11.5, 81.3301)
  line L120 (-35.5, 86.5263) -> (-32.5, 86.5263)
  line L121 (-32.5, 86.5263) -> (-31, 83.9282)
  line L122 (-31, 83.9282) -> (-32.5, 81.3301)
  line L123 (-32.5, 81.3301) -> (-35.5, 81.3301)
  line L124 (-35.5, 81.3301) -> (-37, 83.9282)
  line L125 (-37, 83.9282) -> (-35.5, 86.5263)
  line L126 (-43.5, 81.3301) -> (-45, 83.9282)
  line L127 (-45, 83.9282) -> (-43.5, 86.5263)
  line L128 (-43.5, 86.5263) -> (-40.5, 86.5263)
  line L129 (-40.5, 86.5263) -> (-39, 83.9282)
  line L130 (-39, 83.9282) -> (-40.5, 81.3301)
  line L131 (-40.5, 81.3301) -> (-43.5, 81.3301)
  line L132 (-63.5, 93.4545) -> (-60.5, 93.4545)
  line L133 (-60.5, 93.4545) -> (-59, 90.8564)
  line L134 (-59, 90.8564) -> (-60.5, 88.2583)
  line L135 (-60.5, 88.2583) -> (-63.5, 88.2583)
  line L136 (-63.5, 88.2583) -> (-65, 90.8564)
  line L137 (-65, 90.8564) -> (-63.5, 93.4545)
  line L138 (-47.5, 93.4545) -> (-44.5, 93.4545)
  line L139 (-44.5, 93.4545) -> (-43, 90.8564)
  line L140 (-43, 90.8564) -> (-44.5, 88.2583)
  line L141 (-44.5, 88.2583) -> (-47.5, 88.2583)
  line L142 (-47.5, 88.2583) -> (-49, 90.8564)
  line L143 (-49, 90.8564) -> (-47.5, 93.4545)
  line L144 (-75, 90.8564) -> (-76.5, 88.2583)
  line L145 (-76.5, 88.2583) -> (-79.5, 88.2583)
  line L146 (-79.5, 88.2583) -> (-81, 90.8564)
  line L147 (-81, 90.8564) -> (-79.5, 93.4545)
  line L148 (-79.5, 93.4545) -> (-76.5, 93.4545)
  line L149 (-76.5, 93.4545) -> (-75, 90.8564)
  line L150 (-59.5, 86.5263) -> (-56.5, 86.5263)
  line L151 (-56.5, 86.5263) -> (-55, 83.9282)
  line L152 (-55, 83.9282) -> (-56.5, 81.3301)
  line L153 (-56.5, 81.3301) -> (-59.5, 81.3301)
  line L154 (-59.5, 81.3301) -> (-61, 83.9282)
  line L155 (-61, 83.9282) -> (-59.5, 86.5263)
  line L156 (-75.5, 81.3301) -> (-77, 83.9282)
  line L157 (-77, 83.9282) -> (-75.5, 86.5263)
  line L158 (-75.5, 86.5263) -> (-72.5, 86.5263)
  line L159 (-72.5, 86.5263) -> (-71, 83.9282)
  line L160 (-71, 83.9282) -> (-72.5, 81.3301)
  line L161 (-72.5, 81.3301) -> (-75.5, 81.3301)
  line L162 (-3, 76.8564) -> (-4.5, 74.2583)
  line L163 (-4.5, 74.2583) -> (-7.5, 74.2583)
  line L164 (-7.5, 74.2583) -> (-9, 76.8564)
  line L165 (-9, 76.8564) -> (-7.5, 79.4545)
  line L166 (-7.5, 79.4545) -> (-4.5, 79.4545)
  line L167 (-4.5, 79.4545) -> (-3, 76.8564)
  line L168 (-31.5, 79.4545) -> (-28.5, 79.4545)
  line L169 (-28.5, 79.4545) -> (-27, 76.8564)
  line L170 (-27, 76.8564) -> (-28.5, 74.2583)
  line L171 (-28.5, 74.2583) -> (-31.5, 74.2583)
  line L172 (-31.5, 74.2583) -> (-33, 76.8564)
  line L173 (-33, 76.8564) -> (-31.5, 79.4545)
  line L174 (-15, 69.9282) -> (-16.5, 67.3301)
  line L175 (-16.5, 67.3301) -> (-19.5, 67.3301)
  line L176 (-19.5, 67.3301) -> (-21, 69.9282)
  line L177 (-21, 69.9282) -> (-19.5, 72.5263)
  line L178 (-19.5, 72.5263) -> (-16.5, 72.5263)
  line L179 (-16.5, 72.5263) -> (-15, 69.9282)
  line L180 (-27.5, 72.5263) -> (-24.5, 72.5263)
  line L181 (-24.5, 72.5263) -> (-23, 69.9282)
  line L182 (-23, 69.9282) -> (-24.5, 67.3301)
  line L183 (-24.5, 67.3301) -> (-27.5, 67.3301)
  line L184 (-27.5, 67.3301) -> (-29, 69.9282)
  line L185 (-29, 69.9282) -> (-27.5, 72.5263)
  line L186 (-43.5, 67.3301) -> (-45, 69.9282)
  line L187 (-45, 69.9282) -> (-43.5, 72.5263)
  line L188 (-43.5, 72.5263) -> (-40.5, 72.5263)
  line L189 (-40.5, 72.5263) -> (-39, 69.9282)
  line L190 (-39, 69.9282) -> (-40.5, 67.3301)
  line L191 (-40.5, 67.3301) -> (-43.5, 67.3301)
  line L192 (-63.5, 79.4545) -> (-60.5, 79.4545)
  line L193 (-60.5, 79.4545) -> (-59, 76.8564)
  line L194 (-59, 76.8564) -> (-60.5, 74.2583)
  line L195 (-60.5, 74.2583) -> (-63.5, 74.2583)
  line L196 (-63.5, 74.2583) -> (-65, 76.8564)
  line L197 (-65, 76.8564) -> (-63.5, 79.4545)
  line L198 (-47.5, 79.4545) -> (-44.5, 79.4545)
  line L199 (-44.5, 79.4545) -> (-43, 76.8564)
  line L200 (-43, 76.8564) -> (-44.5, 74.2583)
  line L201 (-44.5, 74.2583) -> (-47.5, 74.2583)
  line L202 (-47.5, 74.2583) -> (-49, 76.8564)
  line L203 (-49, 76.8564) -> (-47.5, 79.4545)
  line L204 (-75, 76.8564) -> (-76.5, 74.2583)
  line L205 (-76.5, 74.2583) -> (-79.5, 74.2583)
  line L206 (-79.5, 74.2583) -> (-81, 76.8564)
  line L207 (-81, 76.8564) -> (-79.5, 79.4545)
  line L208 (-79.5, 79.4545) -> (-76.5, 79.4545)
  line L209 (-76.5, 79.4545) -> (-75, 76.8564)
  line L210 (-59.5, 72.5263) -> (-56.5, 72.5263)
  line L211 (-56.5, 72.5263) -> (-55, 69.9282)
  line L212 (-55, 69.9282) -> (-56.5, 67.3301)
  line L213 (-56.5, 67.3301) -> (-59.5, 67.3301)
  line L214 (-59.5, 67.3301) -> (-61, 69.9282)
  line L215 (-61, 69.9282) -> (-59.5, 72.5263)
  line L216 (-75.5, 67.3301) -> (-77, 69.9282)
  line L217 (-77, 69.9282) -> (-75.5, 72.5263)
  line L218 (-75.5, 72.5263) -> (-72.5, 72.5263)
  line L219 (-72.5, 72.5263) -> (-71, 69.9282)
  line L220 (-71, 69.9282) -> (-72.5, 67.3301)
  line L221 (-72.5, 67.3301) -> (-75.5, 67.3301)
  line L222 (-3, 62.8564) -> (-4.5, 60.2583)
  line L223 (-4.5, 60.2583) -> (-7.5, 60.2583)
  line L224 (-7.5, 60.2583) -> (-9, 62.8564)
  line L225 (-9, 62.8564) -> (-7.5, 65.4545)
  line L226 (-7.5, 65.4545) -> (-4.5, 65.4545)
  line L227 (-4.5, 65.4545) -> (-3, 62.8564)
  line L228 (-31.5, 65.4545) -> (-28.5, 65.4545)
  line L229 (-28.5, 65.4545) -> (-27, 62.8564)
  line L230 (-27, 62.8564) -> (-28.5, 60.2583)
  line L231 (-28.5, 60.2583) -> (-31.5, 60.2583)
  line L232 (-31.5, 60.2583) -> (-33, 62.8564)
  line L233 (-33, 62.8564) -> (-31.5, 65.4545)
  line L234 (-15, 55.9282) -> (-16.5, 53.3301)
  line L235 (-16.5, 53.3301) -> (-19.5, 53.3301)
  line L236 (-19.5, 53.3301) -> (-21, 55.9282)
  line L237 (-21, 55.9282) -> (-19.5, 58.5263)
  line L238 (-19.5, 58.5263) -> (-16.5, 58.5263)
  line L239 (-16.5, 58.5263) -> (-15, 55.9282)
  line L240 (-27.5, 58.5263) -> (-24.5, 58.5263)
  line L241 (-24.5, 58.5263) -> (-23, 55.9282)
  line L242 (-23, 55.9282) -> (-24.5, 53.3301)
  line L243 (-24.5, 53.3301) -> (-27.5, 53.3301)
  line L244 (-27.5, 53.3301) -> (-29, 55.9282)
  line L245 (-29, 55.9282) -> (-27.5, 58.5263)
  line L246 (-43.5, 53.3301) -> (-45, 55.9282)
  line L247 (-45, 55.9282) -> (-43.5, 58.5263)
  line L248 (-43.5, 58.5263) -> (-40.5, 58.5263)
  line L249 (-40.5, 58.5263) -> (-39, 55.9282)
  line L250 (-39, 55.9282) -> (-40.5, 53.3301)
  line L251 (-40.5, 53.3301) -> (-43.5, 53.3301)
  line L252 (-63.5, 65.4545) -> (-60.5, 65.4545)
  line L253 (-60.5, 65.4545) -> (-59, 62.8564)
  line L254 (-59, 62.8564) -> (-60.5, 60.2583)
  line L255 (-60.5, 60.2583) -> (-63.5, 60.2583)
  line L256 (-63.5, 60.2583) -> (-65, 62.8564)
  line L257 (-65, 62.8564) -> (-63.5, 65.4545)
  line L258 (-47.5, 65.4545) -> (-44.5, 65.4545)
  line L259 (-44.5, 65.4545) -> (-43, 62.8564)
  line L260 (-43, 62.8564) -> (-44.5, 60.2583)
  line L261 (-44.5, 60.2583) -> (-47.5, 60.2583)
  line L262 (-47.5, 60.2583) -> (-49, 62.8564)
  line L263 (-49, 62.8564) -> (-47.5, 65.4545)
  line L264 (-75, 62.8564) -> (-76.5, 60.2583)
  line L265 (-76.5, 60.2583) -> (-79.5, 60.2583)
  line L266 (-79.5, 60.2583) -> (-81, 62.8564)
  line L267 (-81, 62.8564) -> (-79.5, 65.4545)
  line L268 (-79.5, 65.4545) -> (-76.5, 65.4545)
  line L269 (-76.5, 65.4545) -> (-75, 62.8564)
  line L270 (-59.5, 58.5263) -> (-56.5, 58.5263)
  line L271 (-56.5, 58.5263) -> (-55, 55.9282)
  line L272 (-55, 55.9282) -> (-56.5, 53.3301)
  line L273 (-56.5, 53.3301) -> (-59.5, 53.3301)
  line L274 (-59.5, 53.3301) -> (-61, 55.9282)
  line L275 (-61, 55.9282) -> (-59.5, 58.5263)
  line L276 (-75.5, 53.3301) -> (-77, 55.9282)
  line L277 (-77, 55.9282) -> (-75.5, 58.5263)
  line L278 (-75.5, 58.5263) -> (-72.5, 58.5263)
  line L279 (-72.5, 58.5263) -> (-71, 55.9282)
  line L280 (-71, 55.9282) -> (-72.5, 53.3301)
  line L281 (-72.5, 53.3301) -> (-75.5, 53.3301)
  line L282 (-3, 48.8564) -> (-4.5, 46.2583)
  line L283 (-4.5, 46.2583) -> (-7.5, 46.2583)
  line L284 (-7.5, 46.2583) -> (-9, 48.8564)
  line L285 (-9, 48.8564) -> (-7.5, 51.4545)
  line L286 (-7.5, 51.4545) -> (-4.5, 51.4545)
  line L287 (-4.5, 51.4545) -> (-3, 48.8564)
  line L288 (-31.5, 51.4545) -> (-28.5, 51.4545)
  line L289 (-28.5, 51.4545) -> (-27, 48.8564)
  line L290 (-27, 48.8564) -> (-28.5, 46.2583)
  line L291 (-28.5, 46.2583) -> (-31.5, 46.2583)
  line L292 (-31.5, 46.2583) -> (-33, 48.8564)
  line L293 (-33, 48.8564) -> (-31.5, 51.4545)
  line L294 (-15, 41.9282) -> (-16.5, 39.3301)
  line L295 (-16.5, 39.3301) -> (-19.5, 39.3301)
  line L296 (-19.5, 39.3301) -> (-21, 41.9282)
  line L297 (-21, 41.9282) -> (-19.5, 44.5263)
  line L298 (-19.5, 44.5263) -> (-16.5, 44.5263)
  line L299 (-16.5, 44.5263) -> (-15, 41.9282)
  line L300 (-27.5, 44.5263) -> (-24.5, 44.5263)
  line L301 (-24.5, 44.5263) -> (-23, 41.9282)
  line L302 (-23, 41.9282) -> (-24.5, 39.3301)
  line L303 (-24.5, 39.3301) -> (-27.5, 39.3301)
  line L304 (-27.5, 39.3301) -> (-29, 41.9282)
  line L305 (-29, 41.9282) -> (-27.5, 44.5263)
  line L306 (-43.5, 39.3301) -> (-45, 41.9282)
  line L307 (-45, 41.9282) -> (-43.5, 44.5263)
  line L308 (-43.5, 44.5263) -> (-40.5, 44.5263)
  line L309 (-40.5, 44.5263) -> (-39, 41.9282)
  line L310 (-39, 41.9282) -> (-40.5, 39.3301)
  line L311 (-40.5, 39.3301) -> (-43.5, 39.3301)
  line L312 (-63.5, 51.4545) -> (-60.5, 51.4545)
  line L313 (-60.5, 51.4545) -> (-59, 48.8564)
  line L314 (-59, 48.8564) -> (-60.5, 46.2583)
  line L315 (-60.5, 46.2583) -> (-63.5, 46.2583)
  line L316 (-63.5, 46.2583) -> (-65, 48.8564)
  line L317 (-65, 48.8564) -> (-63.5, 51.4545)
  line L318 (-47.5, 51.4545) -> (-44.5, 51.4545)
  line L319 (-44.5, 51.4545) -> (-43, 48.8564)
  line L320 (-43, 48.8564) -> (-44.5, 46.2583)
  line L321 (-44.5, 46.2583) -> (-47.5, 46.2583)
  line L322 (-47.5, 46.2583) -> (-49, 48.8564)
  line L323 (-49, 48.8564) -> (-47.5, 51.4545)
  line L324 (-75, 48.8564) -> (-76.5, 46.2583)
  line L325 (-76.5, 46.2583) -> (-79.5, 46.2583)
  line L326 (-79.5, 46.2583) -> (-81, 48.8564)
  line L327 (-81, 48.8564) -> (-79.5, 51.4545)
  line L328 (-79.5, 51.4545) -> (-76.5, 51.4545)
  line L329 (-76.5, 51.4545) -> (-75, 48.8564)
  line L330 (-59.5, 44.5263) -> (-56.5, 44.5263)
  line L331 (-56.5, 44.5263) -> (-55, 41.9282)
  line L332 (-55, 41.9282) -> (-56.5, 39.3301)
  line L333 (-56.5, 39.3301) -> (-59.5, 39.3301)
  line L334 (-59.5, 39.3301) -> (-61, 41.9282)
  line L335 (-61, 41.9282) -> (-59.5, 44.5263)
  line L336 (-75.5, 39.3301) -> (-77, 41.9282)
  line L337 (-77, 41.9282) -> (-75.5, 44.5263)
  line L338 (-75.5, 44.5263) -> (-72.5, 44.5263)
  line L339 (-72.5, 44.5263) -> (-71, 41.9282)
  line L340 (-71, 41.9282) -> (-72.5, 39.3301)
  line L341 (-72.5, 39.3301) -> (-75.5, 39.3301)
  line L342 (-3, 34.8564) -> (-4.5, 32.2583)
  line L343 (-4.5, 32.2583) -> (-7.5, 32.2583)
  line L344 (-7.5, 32.2583) -> (-9, 34.8564)
  line L345 (-9, 34.8564) -> (-7.5, 37.4545)
  line L346 (-7.5, 37.4545) -> (-4.5, 37.4545)
  line L347 (-4.5, 37.4545) -> (-3, 34.8564)
  line L348 (-31.5, 37.4545) -> (-28.5, 37.4545)
  line L349 (-28.5, 37.4545) -> (-27, 34.8564)
  line L350 (-27, 34.8564) -> (-28.5, 32.2583)
  line L351 (-28.5, 32.2583) -> (-31.5, 32.2583)
  line L352 (-31.5, 32.2583) -> (-33, 34.8564)
  line L353 (-33, 34.8564) -> (-31.5, 37.4545)
  line L354 (-15, 27.9282) -> (-16.5, 25.3301)
  line L355 (-16.5, 25.3301) -> (-19.5, 25.3301)
  line L356 (-19.5, 25.3301) -> (-21, 27.9282)
  line L357 (-21, 27.9282) -> (-19.5, 30.5263)
  line L358 (-19.5, 30.5263) -> (-16.5, 30.5263)
  line L359 (-16.5, 30.5263) -> (-15, 27.9282)
  line L360 (-27.5, 30.5263) -> (-24.5, 30.5263)
  line L361 (-24.5, 30.5263) -> (-23, 27.9282)
  line L362 (-23, 27.9282) -> (-24.5, 25.3301)
  line L363 (-24.5, 25.3301) -> (-27.5, 25.3301)
  line L364 (-27.5, 25.3301) -> (-29, 27.9282)
  line L365 (-29, 27.9282) -> (-27.5, 30.5263)
  line L366 (-43.5, 25.3301) -> (-45, 27.9282)
  line L367 (-45, 27.9282) -> (-43.5, 30.5263)
  line L368 (-43.5, 30.5263) -> (-40.5, 30.5263)
  line L369 (-40.5, 30.5263) -> (-39, 27.9282)
  line L370 (-39, 27.9282) -> (-40.5, 25.3301)
  line L371 (-40.5, 25.3301) -> (-43.5, 25.3301)
  line L372 (-63.5, 37.4545) -> (-60.5, 37.4545)
  line L373 (-60.5, 37.4545) -> (-59, 34.8564)
  line L374 (-59, 34.8564) -> (-60.5, 32.2583)
  line L375 (-60.5, 32.2583) -> (-63.5, 32.2583)
  line L376 (-63.5, 32.2583) -> (-65, 34.8564)
  line L377 (-65, 34.8564) -> (-63.5, 37.4545)
  line L378 (-47.5, 37.4545) -> (-44.5, 37.4545)
  line L379 (-44.5, 37.4545) -> (-43, 34.8564)
  line L380 (-43, 34.8564) -> (-44.5, 32.2583)
  line L381 (-44.5, 32.2583) -> (-47.5, 32.2583)
  line L382 (-47.5, 32.2583) -> (-49, 34.8564)
  line L383 (-49, 34.8564) -> (-47.5, 37.4545)
  line L384 (-75, 34.8564) -> (-76.5, 32.2583)
  line L385 (-76.5, 32.2583) -> (-79.5, 32.2583)
  line L386 (-79.5, 32.2583) -> (-81, 34.8564)
  line L387 (-81, 34.8564) -> (-79.5, 37.4545)
  line L388 (-79.5, 37.4545) -> (-76.5, 37.4545)
  line L389 (-76.5, 37.4545) -> (-75, 34.8564)
  line L390 (-59.5, 30.5263) -> (-56.5, 30.5263)
  line L391 (-56.5, 30.5263) -> (-55, 27.9282)
  line L392 (-55, 27.9282) -> (-56.5, 25.3301)
  line L393 (-56.5, 25.3301) -> (-59.5, 25.3301)
  line L394 (-59.5, 25.3301) -> (-61, 27.9282)
  line L395 (-61, 27.9282) -> (-59.5, 30.5263)
  line L396 (-75.5, 25.3301) -> (-77, 27.9282)
  line L397 (-77, 27.9282) -> (-75.5, 30.5263)
  line L398 (-75.5, 30.5263) -> (-72.5, 30.5263)
  line L399 (-72.5, 30.5263) -> (-71, 27.9282)
  line L400 (-71, 27.9282) -> (-72.5, 25.3301)
  line L401 (-72.5, 25.3301) -> (-75.5, 25.3301)
  line L402 (-7.5, 18.2583) -> (-9, 20.8564)
  line L403 (-9, 20.8564) -> (-7.5, 23.4545)
  line L404 (-7.5, 23.4545) -> (-4.5, 23.4545)
  line L405 (-4.5, 23.4545) -> (-3, 20.8564)
  line L406 (-3, 20.8564) -> (-4.5, 18.2583)
  line L407 (-4.5, 18.2583) -> (-7.5, 18.2583)
  line L408 (-71.5, 18.2583) -> (-73, 20.8564)
  line L409 (-73, 20.8564) -> (-71.5, 23.4545)
  line L410 (-71.5, 23.4545) -> (-68.5, 23.4545)
  line L411 (-68.5, 23.4545) -> (-67, 20.8564)
  line L412 (-67, 20.8564) -> (-68.5, 18.2583)
  line L413 (-68.5, 18.2583) -> (-71.5, 18.2583)
  line L414 (-55.5, 18.2583) -> (-57, 20.8564)
  line L415 (-57, 20.8564) -> (-55.5, 23.4545)
  line L416 (-55.5, 23.4545) -> (-52.5, 23.4545)
  line L417 (-52.5, 23.4545) -> (-51, 20.8564)
  line L418 (-51, 20.8564) -> (-52.5, 18.2583)
  line L419 (-52.5, 18.2583) -> (-55.5, 18.2583)
  line L420 (-39.5, 18.2583) -> (-41, 20.8564)
  line L421 (-41, 20.8564) -> (-39.5, 23.4545)
  line L422 (-39.5, 23.4545) -> (-36.5, 23.4545)
  line L423 (-36.5, 23.4545) -> (-35, 20.8564)
  line L424 (-35, 20.8564) -> (-36.5, 18.2583)
  line L425 (-36.5, 18.2583) -> (-39.5, 18.2583)
  line L426 (-23.5, 18.2583) -> (-25, 20.8564)
  line L427 (-25, 20.8564) -> (-23.5, 23.4545)
  line L428 (-23.5, 23.4545) -> (-20.5, 23.4545)
  line L429 (-20.5, 23.4545) -> (-19, 20.8564)
  line L430 (-19, 20.8564) -> (-20.5, 18.2583)
  line L431 (-20.5, 18.2583) -> (-23.5, 18.2583)
  line L432 (-83.5, 11.3301) -> (-85, 13.9282)
  line L433 (-85, 13.9282) -> (-83.5, 16.5263)
  line L434 (-83.5, 16.5263) -> (-80.5, 16.5263)
  line L435 (-80.5, 16.5263) -> (-79, 13.9282)
  line L436 (-79, 13.9282) -> (-80.5, 11.3301)
  line L437 (-80.5, 11.3301) -> (-83.5, 11.3301)
  line L438 (-67.5, 11.3301) -> (-69, 13.9282)
  line L439 (-69, 13.9282) -> (-67.5, 16.5263)
  line L440 (-67.5, 16.5263) -> (-64.5, 16.5263)
  line L441 (-64.5, 16.5263) -> (-63, 13.9282)
  line L442 (-63, 13.9282) -> (-64.5, 11.3301)
  line L443 (-64.5, 11.3301) -> (-67.5, 11.3301)
  line L444 (-51.5, 11.3301) -> (-53, 13.9282)
  line L445 (-53, 13.9282) -> (-51.5, 16.5263)
  line L446 (-51.5, 16.5263) -> (-48.5, 16.5263)
  line L447 (-48.5, 16.5263) -> (-47, 13.9282)
  line L448 (-47, 13.9282) -> (-48.5, 11.3301)
  line L449 (-48.5, 11.3301) -> (-51.5, 11.3301)
  line L450 (-35.5, 11.3301) -> (-37, 13.9282)
  line L451 (-37, 13.9282) -> (-35.5, 16.5263)
  line L452 (-35.5, 16.5263) -> (-32.5, 16.5263)
  line L453 (-32.5, 16.5263) -> (-31, 13.9282)
  line L454 (-31, 13.9282) -> (-32.5, 11.3301)
  line L455 (-32.5, 11.3301) -> (-35.5, 11.3301)
  line L456 (-19.5, 11.3301) -> (-21, 13.9282)
  line L457 (-21, 13.9282) -> (-19.5, 16.5263)
  line L458 (-19.5, 16.5263) -> (-16.5, 16.5263)
  line L459 (-16.5, 16.5263) -> (-15, 13.9282)
  line L460 (-15, 13.9282) -> (-16.5, 11.3301)
  line L461 (-16.5, 11.3301) -> (-19.5, 11.3301)
  line L462 (-63.5, 4.4019) -> (-65, 7)
  line L463 (-65, 7) -> (-63.5, 9.5981)
  line L464 (-63.5, 9.5981) -> (-60.5, 9.5981)
  line L465 (-60.5, 9.5981) -> (-59, 7)
  line L466 (-59, 7) -> (-60.5, 4.4019)
  line L467 (-60.5, 4.4019) -> (-63.5, 4.4019)
  line L468 (-47.5, 4.4019) -> (-49, 7)
  line L469 (-49, 7) -> (-47.5, 9.5981)
  line L470 (-47.5, 9.5981) -> (-44.5, 9.5981)
  line L471 (-44.5, 9.5981) -> (-43, 7)
  line L472 (-43, 7) -> (-44.5, 4.4019)
  line L473 (-44.5, 4.4019) -> (-47.5, 4.4019)
  line L474 (-31.5, 4.4019) -> (-33, 7)
  line L475 (-33, 7) -> (-31.5, 9.5981)
  line L476 (-31.5, 9.5981) -> (-28.5, 9.5981)
  line L477 (-28.5, 9.5981) -> (-27, 7)
  line L478 (-27, 7) -> (-28.5, 4.4019)